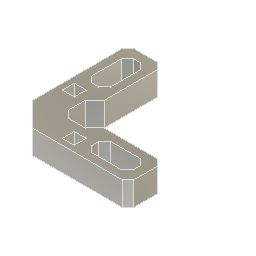
уголок (Autodesk Fusion 360 design; units mm, degrees)
Autodesk Fusion 360 part; units mm, degrees
sketch "Sketch1" plane through (0, 0, 0) normal (0, 0, 1) x (1, 0, 0)
  line L0 (-30, 70) -> (-30, -10)
  line L1 (70, -30) -> (-10, -30)
  line L2 (0, 70) -> (-30, 70)
  line L3 (70, 0) -> (70, -30)
  line L4 (-10, -30) -> (-30, -10)
  line L5 (5, -15) -> (-15, 5)
  line L6 (-15, 5) -> (0, 20)
  line L7 (5, -15) -> (20, 0)
  line L8 (0, 70) -> (0, 0)
  line L9 (0, 0) -> (70, 0)
  line L10 (62.5, -7) -> (27.5, -7)
  line L11 (27.5, -7) -> (27.5, -23)
  line L12 (27.5, -23) -> (62.5, -23)
  line L13 (62.5, -23) -> (62.5, -7)
  line L14 (62.5, -7) -> (27.5, -23) construction
  line L15 (27.5, -7) -> (62.5, -23) construction
  line L16 (-7, 62.5) -> (-23, 62.5)
  line L17 (-23, 62.5) -> (-23, 27.5)
  line L18 (-23, 27.5) -> (-7, 27.5)
  line L19 (-7, 27.5) -> (-7, 62.5)
  line L20 (-7, 62.5) -> (-23, 27.5) construction
  line L21 (-23, 62.5) -> (-7, 27.5) construction
  line L22 (-25, 10) -> (-15, 10)
  line L23 (-15, 10) -> (-15, 20)
  line L24 (-15, 20) -> (-25, 20)
  line L25 (-25, 20) -> (-25, 10)
  line L26 (-25, 10) -> (-15, 20) construction
  line L27 (-15, 10) -> (-25, 20) construction
  line L28 (10, -25) -> (20, -25)
  line L29 (20, -25) -> (20, -15)
  line L30 (20, -15) -> (10, -15)
  line L31 (10, -15) -> (10, -25)
  line L32 (10, -25) -> (20, -15) construction
  line L33 (20, -25) -> (10, -15) construction
  point P0 (45, -15)
  point P1 (-15, 45)
  point P2 (-20, 15)
  point P3 (15, -20)
  dimension "d15" = 35
  dimension "d16" = 16
  dimension "d17" = 16
  dimension "d18" = 35
  constraint coincident L8.end L9.start
  constraint parallel L4 L5
  constraint perpendicular L5 L6
  constraint perpendicular L5 L7
  constraint perpendicular L2 L8
  constraint perpendicular L3 L9
  constraint coincident L7.end L9
  constraint coincident L6.end L8
  constraint horizontal L10
  constraint perpendicular L10 L11
  constraint parallel L10 L12
  constraint parallel L11 L13
  constraint coincident L14 P0
  constraint coincident L15 P0
  constraint horizontal L16
  constraint perpendicular L16 L17
  constraint parallel L16 L18
  constraint parallel L17 L19
  constraint coincident L20 P1
  constraint coincident L21 P1
  constraint horizontal L22
  constraint perpendicular L22 L23
  constraint parallel L22 L24
  constraint parallel L23 L25
  constraint coincident L26 P2
  constraint coincident L27 P2
  constraint horizontal L28
  constraint perpendicular L28 L29
  constraint parallel L28 L30
  constraint parallel L29 L31
  constraint coincident L32 P3
  constraint coincident L33 P3
  measures "d15" distance of L11.end L12.end
  measures "d16" distance of L10.end L11.end
  measures "d17" distance of L17.end L18.end
  measures "d18" distance of L16.end L17.end
extrude "Extrude1" add sketch "Sketch1" along normal blind 20 contours L0 L1 L2 L3 L4 L5 L6 L7 L8 L9
chamfer "Chamfer1" distance 10 angle 45 2 edges at (-15, 5, 10) (5, -15, 10)
chamfer "Chamfer3" distance 5 angle 45 8 edges at (-23, 62.5, 10) (-7, 62.5, 10) (-7, 27.5, 10) (-23, 27.5, 10) (27.5, -23, 10) (27.5, -7, 10) (62.5, -7, 10) (62.5, -23, 10)
chamfer "Chamfer4" distance 5 angle 45 4 edges at (-30, 70, 10) (0, 70, 10) (70, 0, 10) (70, -30, 10)
